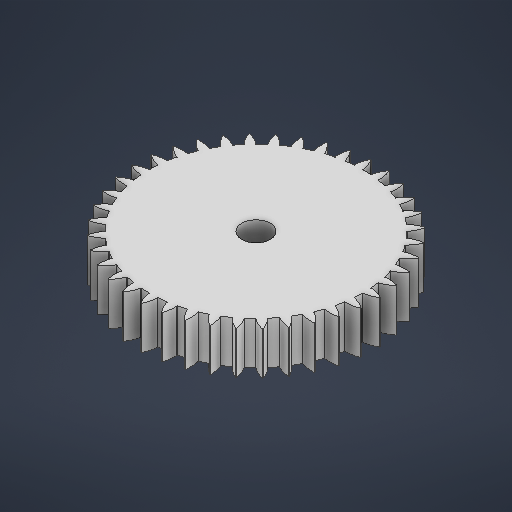
# Autodesk Inventor part: 80mm_40N_Gear
Saved by Autodesk Inventor 2026.2 (Build 302298000, 298)
## iProperties
Created: 2025-12-19
Part Number: 80mm_40N_Gear
Material: Generic
Document SubType Name: Modeling
Designer: Cobble
Density: 1 g/cm^3
Appearance: Default
Author: Cobble
Autodesk Inventor part; units mm, degrees
ref_plane "YZ Plane" through (0, 0, 0) normal (1, 0, 0) x (0, 1, 0)
ref_plane "XZ Plane" through (0, 0, 0) normal (0, 1, 0) x (-1, 0, 0)
ref_plane "XY Plane" through (0, 0, 0) normal (0, 0, 1) x (1, 0, 0)
sketch "Sketch1" plane through (0, 0, 0) normal (0, 0, 1) x (1, 0, 0)
  circle A0 centre (0, 0) radius 40
  circle A1 centre (0, 0) radius 42
  circle A2 centre (0, 0) radius 37.5
  circle A3 centre (0, 0) radius 37.5877 construction
  line L0 (0, 0) -> (0, 42) construction
  line L1 (0, 0) -> (-6.5702, 41.4829) construction
  line L2 (0, 0) -> (-12.9787, 39.9444) construction
  line L3 (0, 0) -> (-19.0676, 37.4223) construction
  line L4 (0, 0) -> (-24.687, 33.9787) construction
  line L5 (0, 0) -> (-29.6985, 29.6985) construction
  line L6 (0, 0) -> (-33.9787, 24.687) construction
  line L7 (0, 0) -> (-37.4223, 19.0676) construction
  line L8 (0, 0) -> (-39.9444, 12.9787) construction
  line L9 (0, 0) -> (-41.4829, 6.5702) construction
  line L10 (0, 0) -> (-42, 0) construction
  line L11 (0, 0) -> (-41.4829, -6.5702) construction
  line L12 (0, 0) -> (-39.9444, -12.9787) construction
  line L13 (0, 0) -> (-37.4223, -19.0676) construction
  line L14 (0, 0) -> (-33.9787, -24.687) construction
  line L15 (0, 0) -> (-29.6985, -29.6985) construction
  line L16 (0, 0) -> (-24.687, -33.9787) construction
  line L17 (0, 0) -> (-19.0676, -37.4223) construction
  line L18 (0, 0) -> (-12.9787, -39.9444) construction
  line L19 (0, 0) -> (-6.5702, -41.4829) construction
  line L20 (0, 0) -> (0, -42) construction
  line L21 (0, 0) -> (6.5702, -41.4829) construction
  line L22 (0, 0) -> (12.9787, -39.9444) construction
  line L23 (0, 0) -> (19.0676, -37.4223) construction
  line L24 (0, 0) -> (24.687, -33.9787) construction
  line L25 (0, 0) -> (29.6985, -29.6985) construction
  line L26 (0, 0) -> (33.9787, -24.687) construction
  line L27 (0, 0) -> (37.4223, -19.0676) construction
  line L28 (0, 0) -> (39.9444, -12.9787) construction
  line L29 (0, 0) -> (41.4829, -6.5702) construction
  line L30 (0, 0) -> (42, 0) construction
  line L31 (0, 0) -> (41.4829, 6.5702) construction
  line L32 (0, 0) -> (39.9444, 12.9787) construction
  line L33 (0, 0) -> (37.4223, 19.0676) construction
  line L34 (0, 0) -> (33.9787, 24.687) construction
  line L35 (0, 0) -> (29.6985, 29.6985) construction
  line L36 (0, 0) -> (24.687, 33.9787) construction
  line L37 (0, 0) -> (19.0676, 37.4223) construction
  line L38 (0, 0) -> (12.9787, 39.9444) construction
  line L39 (0, 0) -> (6.5702, 41.4829) construction
  line L40 (-5.88, 37.1249) -> (-0.0487, 38.0485) construction
  line L41 (-11.6152, 35.748) -> (-0.3852, 39.3969) construction
  line L42 (-17.0645, 33.4909) -> (-1.283, 41.532) construction
  line L43 (-22.0935, 30.4091) -> (-2.9878, 44.2902) construction
  line L44 (-26.5785, 26.5785) -> (-5.7047, 47.4523) construction
  line L45 (0, 0) -> (3.1384, 39.8767) construction
  line L46 (0, 0) -> (40, 0) construction
  line L47 (0, 0) -> (-3.1384, 39.8767) construction
  line L48 (0, 0) -> (-9.3378, 38.8948) construction
  line L49 (0, 0) -> (-15.3073, 36.9552) construction
  line L50 (0, 0) -> (-20.8999, 34.1056) construction
  line L51 (0, 0) -> (-25.9779, 30.4162) construction
  line L52 (0, 0) -> (-30.4162, 25.9779) construction
  line L53 (0, 0) -> (-34.1056, 20.8999) construction
  line L54 (0, 0) -> (-36.9552, 15.3073) construction
  line L55 (0, 0) -> (-38.8948, 9.3378) construction
  line L56 (0, 0) -> (-39.8767, 3.1384) construction
  line L57 (0, 0) -> (-39.8767, -3.1384) construction
  line L58 (0, 0) -> (-38.8948, -9.3378) construction
  line L59 (0, 0) -> (-36.9552, -15.3073) construction
  line L60 (0, 0) -> (-34.1056, -20.8999) construction
  line L61 (0, 0) -> (-30.4162, -25.9779) construction
  line L62 (0, 0) -> (-25.9779, -30.4162) construction
  line L63 (0, 0) -> (-20.8999, -34.1056) construction
  line L64 (0, 0) -> (-15.3073, -36.9552) construction
  line L65 (0, 0) -> (-9.3378, -38.8948) construction
  line L66 (0, 0) -> (-3.1384, -39.8767) construction
  line L67 (0, 0) -> (3.1384, -39.8767) construction
  line L68 (0, 0) -> (9.3378, -38.8948) construction
  line L69 (0, 0) -> (15.3073, -36.9552) construction
  line L70 (0, 0) -> (20.8999, -34.1056) construction
  line L71 (0, 0) -> (25.9779, -30.4162) construction
  line L72 (0, 0) -> (30.4162, -25.9779) construction
  line L73 (0, 0) -> (34.1056, -20.8999) construction
  line L74 (0, 0) -> (36.9552, -15.3073) construction
  line L75 (0, 0) -> (38.8948, -9.3378) construction
  line L76 (0, 0) -> (39.8767, -3.1384) construction
  line L77 (0, 0) -> (39.8767, 3.1384) construction
  line L78 (0, 0) -> (38.8948, 9.3378) construction
  line L79 (0, 0) -> (36.9552, 15.3073) construction
  line L80 (0, 0) -> (34.1056, 20.8999) construction
  line L81 (0, 0) -> (30.4162, 25.9779) construction
  line L82 (0, 0) -> (25.9779, 30.4162) construction
  line L83 (0, 0) -> (20.8999, 34.1056) construction
  line L84 (0, 0) -> (15.3073, 36.9552) construction
  line L85 (0, 0) -> (9.3378, 38.8948) construction
  line L86 (2.9491, 37.4718) -> (-2.9367, 37.9351) construction
  line L87 (8.7747, 36.5492) -> (-2.7071, 39.3057) construction
  line L88 (14.3842, 34.7265) -> (-1.9796, 41.5046) construction
  line L89 (19.6395, 32.0488) -> (-0.4964, 44.3881) construction
  line L90 (24.4113, 28.5819) -> (1.9641, 47.7536) construction
  spline S0 degree 4 poles (0, 37.5877) (0.0049, 37.8732) (-0.3682, 40.1269) (-1.7488, 42.8109) (-4.0108, 45.8093) (-5.7047, 47.4523) knots 0 0 0 0 0 0.384274 1 1 1 1 1
  spline S1 degree 4 poles (-2.9491, 37.4718) (-2.9764, 37.756) (-2.7812, 40.0321) (-1.6155, 42.8162) (0.4043, 45.9828) (1.9641, 47.7536) knots 0 0 0 0 0 0.384274 1 1 1 1 1
  line L91 (0, 37.5877) -> (0, 37.5)
  line L92 (-2.9491, 37.4718) -> (-2.9422, 37.3844)
  line L93 (-30.4091, 22.0935) -> (-13.0577, 45.9757) construction
  spline S2 degree 4 poles (-5.88, 37.1249) (-5.9198, 37.4076) (-6.6409, 39.5753) (-8.4244, 42.0103) (-11.1275, 44.6179) (-13.0577, 45.9757) knots 0 0 0 0 0 0.384274 1 1 1 1 1
  spline S3 degree 4 poles (-8.7747, 36.5492) (-8.8461, 36.8256) (-9.0094, 39.1042) (-8.2935, 42.0363) (-6.794, 45.4799) (-5.5304, 47.4729) knots 0 0 0 0 0 0.384274 1 1 1 1 1
  line L94 (-5.88, 37.1249) -> (-5.8663, 37.0383)
  line L95 (-8.7747, 36.5492) -> (-8.7542, 36.4639)
  line L96 (-33.4909, 17.0645) -> (-20.0891, 43.367) construction
  spline S4 degree 4 poles (-11.6152, 35.748) (-11.6988, 36.021) (-12.7501, 38.0492) (-14.8925, 40.1752) (-17.9703, 42.3278) (-20.0891, 43.367) knots 0 0 0 0 0 0.384274 1 1 1 1 1
  spline S5 degree 4 poles (-14.3842, 34.7265) (-14.4979, 34.9884) (-15.0157, 37.2134) (-14.7674, 40.2214) (-13.825, 43.8571) (-12.8887, 46.0233) knots 0 0 0 0 0 0.384274 1 1 1 1 1
  line L97 (-11.6152, 35.748) -> (-11.5881, 35.6646)
  line L98 (-14.3842, 34.7265) -> (-14.3506, 34.6455)
  line L99 (-35.748, 11.6152) -> (-26.6258, 39.6904) construction
  spline S6 degree 4 poles (-17.0645, 33.4909) (-17.1897, 33.7475) (-18.5453, 35.5862) (-20.9939, 37.3509) (-24.3706, 38.9955) (-26.6258, 39.6904) knots 0 0 0 0 0 0.384274 1 1 1 1 1
  spline S7 degree 4 poles (-19.6395, 32.0488) (-19.7928, 32.2896) (-20.6523, 34.4062) (-20.8776, 37.4161) (-20.5156, 41.1545) (-19.9297, 43.4405) knots 0 0 0 0 0 0.384274 1 1 1 1 1
  line L100 (-17.0645, 33.4909) -> (-17.0246, 33.4127)
  line L101 (-19.6395, 32.0488) -> (-19.5937, 31.974)
  line L102 (-37.1249, 5.88) -> (-32.507, 35.0366) construction
  spline S8 degree 4 poles (-22.0935, 30.4091) (-22.2573, 30.6429) (-23.8839, 32.2469) (-26.5784, 33.6069) (-30.1708, 34.703) (-32.507, 35.0366) knots 0 0 0 0 0 0.384274 1 1 1 1 1
  spline S9 degree 4 poles (-24.4113, 28.5819) (-24.6004, 28.7958) (-25.7803, 30.7519) (-26.4737, 33.6894) (-26.7009, 37.4385) (-26.4799, 39.7879) knots 0 0 0 0 0 0.384274 1 1 1 1 1
  line L103 (-22.0935, 30.4091) -> (-22.0419, 30.3381)
  line L104 (-24.4113, 28.5819) -> (-24.3543, 28.5152)
  line L105 (-37.5877, 0) -> (-37.5877, 29.52) construction
  spline S10 degree 4 poles (-26.5785, 26.5785) (-26.7769, 26.7838) (-28.6344, 28.1136) (-31.5085, 29.0353) (-35.2281, 29.556) (-37.5877, 29.52) knots 0 0 0 0 0 0.384274 1 1 1 1 1
  spline S11 degree 4 poles (-28.5819, 24.4113) (-28.8022, 24.5929) (-30.2736, 26.3404) (-31.4179, 29.1333) (-32.2289, 32.8006) (-32.3781, 35.1557) knots 0 0 0 0 0 0.384274 1 1 1 1 1
  line L106 (-26.5785, 26.5785) -> (-26.5165, 26.5165)
  line L107 (-28.5819, 24.4113) -> (-28.5152, 24.3543)
  line L108 (-37.1249, -5.88) -> (-41.7429, 23.2765) construction
  spline S12 degree 4 poles (-30.4091, 22.0935) (-30.6372, 22.2652) (-32.6798, 23.2881) (-35.6627, 23.7488) (-39.418, 23.6813) (-41.7429, 23.2765) knots 0 0 0 0 0 0.384274 1 1 1 1 1
  spline S13 degree 4 poles (-32.0488, 19.6395) (-32.2947, 19.7845) (-34.0214, 21.2802) (-35.5886, 23.8597) (-36.9632, 27.355) (-37.479, 29.6578) knots 0 0 0 0 0 0.384274 1 1 1 1 1
  line L109 (-30.4091, 22.0935) -> (-30.3381, 22.0419)
  line L110 (-32.0488, 19.6395) -> (-31.974, 19.5937)
  line L111 (-35.748, -11.6152) -> (-44.8702, 16.4599) construction
  spline S14 degree 4 poles (-33.4909, 17.0645) (-33.743, 17.1984) (-35.9205, 17.8891) (-38.9388, 17.8776) (-42.6372, 17.2234) (-44.8702, 16.4599) knots 0 0 0 0 0 0.384274 1 1 1 1 1
  spline S15 degree 4 poles (-34.7265, 14.3842) (-34.9921, 14.4889) (-36.9315, 15.6961) (-38.8829, 17.9987) (-40.7874, 21.2359) (-41.6571, 23.4297) knots 0 0 0 0 0 0.384274 1 1 1 1 1
  line L112 (-33.4909, 17.0645) -> (-33.4127, 17.0246)
  line L113 (-34.7265, 14.3842) -> (-34.6455, 14.3506)
  line L114 (-33.4909, -17.0645) -> (-46.8927, 9.2381) construction
  spline S16 degree 4 poles (-35.748, 11.6152) (-36.018, 11.7081) (-38.2768, 12.0497) (-41.256, 11.5661) (-44.8066, 10.3414) (-46.8927, 9.2381) knots 0 0 0 0 0 0.384274 1 1 1 1 1
  spline S17 degree 4 poles (-36.5492, 8.7747) (-36.8279, 8.8366) (-38.9322, 9.7255) (-41.2198, 11.6945) (-43.6073, 14.5939) (-44.8095, 16.6246) knots 0 0 0 0 0 0.384274 1 1 1 1 1
  line L115 (-35.748, 11.6152) -> (-35.6646, 11.5881)
  line L116 (-36.5492, 8.7747) -> (-36.4639, 8.7542)
  line L117 (-30.4091, -22.0935) -> (-47.7605, 1.7887) construction
  spline S18 degree 4 poles (-37.1249, 5.88) (-37.4061, 5.9295) (-39.6905, 5.9135) (-42.5574, 4.9699) (-45.8727, 3.2048) (-47.7605, 1.7887) knots 0 0 0 0 0 0.384274 1 1 1 1 1
  spline S19 degree 4 poles (-37.4718, 2.9491) (-37.7568, 2.9666) (-39.9743, 3.5154) (-42.5418, 5.1023) (-45.3534, 7.5926) (-46.8584, 9.4102) knots 0 0 0 0 0 0.384274 1 1 1 1 1
  line L118 (-37.1249, 5.88) -> (-37.0383, 5.8663)
  line L119 (-37.4718, 2.9491) -> (-37.3844, 2.9422)
  line L120 (-26.5785, -26.5785) -> (-47.4523, -5.7047) construction
  spline S20 degree 4 poles (-37.5877, 0) (-37.8732, 0.0049) (-40.1269, -0.3682) (-42.8109, -1.7488) (-45.8093, -4.0108) (-47.4523, -5.7047) knots 0 0 0 0 0 0.384274 1 1 1 1 1
  spline S21 degree 4 poles (-37.4718, -2.9491) (-37.756, -2.9764) (-40.0321, -2.7812) (-42.8162, -1.6155) (-45.9828, 0.4043) (-47.7536, 1.9641) knots 0 0 0 0 0 0.384274 1 1 1 1 1
  line L121 (-37.5877, 0) -> (-37.5, 0)
  line L122 (-37.4718, -2.9491) -> (-37.3844, -2.9422)
  line L123 (-22.0935, -30.4091) -> (-45.9757, -13.0577) construction
  spline S22 degree 4 poles (-37.1249, -5.88) (-37.4076, -5.9198) (-39.5753, -6.6409) (-42.0103, -8.4244) (-44.6179, -11.1275) (-45.9757, -13.0577) knots 0 0 0 0 0 0.384274 1 1 1 1 1
  spline S23 degree 4 poles (-36.5492, -8.7747) (-36.8256, -8.8461) (-39.1042, -9.0094) (-42.0363, -8.2935) (-45.4799, -6.794) (-47.4729, -5.5304) knots 0 0 0 0 0 0.384274 1 1 1 1 1
  line L124 (-37.1249, -5.88) -> (-37.0383, -5.8663)
  line L125 (-36.5492, -8.7747) -> (-36.4639, -8.7542)
  line L126 (-17.0645, -33.4909) -> (-43.367, -20.0891) construction
  spline S24 degree 4 poles (-35.748, -11.6152) (-36.021, -11.6988) (-38.0492, -12.7501) (-40.1752, -14.8925) (-42.3278, -17.9703) (-43.367, -20.0891) knots 0 0 0 0 0 0.384274 1 1 1 1 1
  spline S25 degree 4 poles (-34.7265, -14.3842) (-34.9884, -14.4979) (-37.2134, -15.0157) (-40.2214, -14.7674) (-43.8571, -13.825) (-46.0233, -12.8887) knots 0 0 0 0 0 0.384274 1 1 1 1 1
  line L127 (-35.748, -11.6152) -> (-35.6646, -11.5881)
  line L128 (-34.7265, -14.3842) -> (-34.6455, -14.3506)
  line L129 (-11.6152, -35.748) -> (-39.6904, -26.6258) construction
  spline S26 degree 4 poles (-33.4909, -17.0645) (-33.7475, -17.1897) (-35.5862, -18.5453) (-37.3509, -20.9939) (-38.9955, -24.3706) (-39.6904, -26.6258) knots 0 0 0 0 0 0.384274 1 1 1 1 1
  spline S27 degree 4 poles (-32.0488, -19.6395) (-32.2896, -19.7928) (-34.4062, -20.6523) (-37.4161, -20.8776) (-41.1545, -20.5156) (-43.4405, -19.9297) knots 0 0 0 0 0 0.384274 1 1 1 1 1
  line L130 (-33.4909, -17.0645) -> (-33.4127, -17.0246)
  line L131 (-32.0488, -19.6395) -> (-31.974, -19.5937)
  line L132 (-5.88, -37.1249) -> (-35.0366, -32.507) construction
  spline S28 degree 4 poles (-30.4091, -22.0935) (-30.6429, -22.2573) (-32.2469, -23.8839) (-33.6069, -26.5784) (-34.703, -30.1708) (-35.0366, -32.507) knots 0 0 0 0 0 0.384274 1 1 1 1 1
  spline S29 degree 4 poles (-28.5819, -24.4113) (-28.7958, -24.6004) (-30.7519, -25.7803) (-33.6894, -26.4737) (-37.4385, -26.7009) (-39.7879, -26.4799) knots 0 0 0 0 0 0.384274 1 1 1 1 1
  line L133 (-30.4091, -22.0935) -> (-30.3381, -22.0419)
  line L134 (-28.5819, -24.4113) -> (-28.5152, -24.3543)
  line L135 (0, -37.5877) -> (-29.52, -37.5877) construction
  spline S30 degree 4 poles (-26.5785, -26.5785) (-26.7838, -26.7769) (-28.1136, -28.6344) (-29.0353, -31.5085) (-29.556, -35.2281) (-29.52, -37.5877) knots 0 0 0 0 0 0.384274 1 1 1 1 1
  spline S31 degree 4 poles (-24.4113, -28.5819) (-24.5929, -28.8022) (-26.3404, -30.2736) (-29.1333, -31.4179) (-32.8006, -32.2289) (-35.1557, -32.3781) knots 0 0 0 0 0 0.384274 1 1 1 1 1
  line L136 (-26.5785, -26.5785) -> (-26.5165, -26.5165)
  line L137 (-24.4113, -28.5819) -> (-24.3543, -28.5152)
  line L138 (5.88, -37.1249) -> (-23.2765, -41.7429) construction
  spline S32 degree 4 poles (-22.0935, -30.4091) (-22.2652, -30.6372) (-23.2881, -32.6798) (-23.7488, -35.6627) (-23.6813, -39.418) (-23.2765, -41.7429) knots 0 0 0 0 0 0.384274 1 1 1 1 1
  spline S33 degree 4 poles (-19.6395, -32.0488) (-19.7845, -32.2947) (-21.2802, -34.0214) (-23.8597, -35.5886) (-27.355, -36.9632) (-29.6578, -37.479) knots 0 0 0 0 0 0.384274 1 1 1 1 1
  line L139 (-22.0935, -30.4091) -> (-22.0419, -30.3381)
  line L140 (-19.6395, -32.0488) -> (-19.5937, -31.974)
  line L141 (11.6152, -35.748) -> (-16.4599, -44.8702) construction
  spline S34 degree 4 poles (-17.0645, -33.4909) (-17.1984, -33.743) (-17.8891, -35.9205) (-17.8776, -38.9388) (-17.2234, -42.6372) (-16.4599, -44.8702) knots 0 0 0 0 0 0.384274 1 1 1 1 1
  spline S35 degree 4 poles (-14.3842, -34.7265) (-14.4889, -34.9921) (-15.6961, -36.9315) (-17.9987, -38.8829) (-21.2359, -40.7874) (-23.4297, -41.6571) knots 0 0 0 0 0 0.384274 1 1 1 1 1
  line L142 (-17.0645, -33.4909) -> (-17.0246, -33.4127)
  line L143 (-14.3842, -34.7265) -> (-14.3506, -34.6455)
  line L144 (17.0645, -33.4909) -> (-9.2381, -46.8927) construction
  spline S36 degree 4 poles (-11.6152, -35.748) (-11.7081, -36.018) (-12.0497, -38.2768) (-11.5661, -41.256) (-10.3414, -44.8066) (-9.2381, -46.8927) knots 0 0 0 0 0 0.384274 1 1 1 1 1
  spline S37 degree 4 poles (-8.7747, -36.5492) (-8.8366, -36.8279) (-9.7255, -38.9322) (-11.6945, -41.2198) (-14.5939, -43.6073) (-16.6246, -44.8095) knots 0 0 0 0 0 0.384274 1 1 1 1 1
  line L145 (-11.6152, -35.748) -> (-11.5881, -35.6646)
  line L146 (-8.7747, -36.5492) -> (-8.7542, -36.4639)
  line L147 (22.0935, -30.4091) -> (-1.7887, -47.7605) construction
  spline S38 degree 4 poles (-5.88, -37.1249) (-5.9295, -37.4061) (-5.9135, -39.6905) (-4.9699, -42.5574) (-3.2048, -45.8727) (-1.7887, -47.7605) knots 0 0 0 0 0 0.384274 1 1 1 1 1
  spline S39 degree 4 poles (-2.9491, -37.4718) (-2.9666, -37.7568) (-3.5154, -39.9743) (-5.1023, -42.5418) (-7.5926, -45.3534) (-9.4102, -46.8584) knots 0 0 0 0 0 0.384274 1 1 1 1 1
  line L148 (-5.88, -37.1249) -> (-5.8663, -37.0383)
  line L149 (-2.9491, -37.4718) -> (-2.9422, -37.3844)
  line L150 (26.5785, -26.5785) -> (5.7047, -47.4523) construction
  spline S40 degree 4 poles (0, -37.5877) (-0.0049, -37.8732) (0.3682, -40.1269) (1.7488, -42.8109) (4.0108, -45.8093) (5.7047, -47.4523) knots 0 0 0 0 0 0.384274 1 1 1 1 1
  spline S41 degree 4 poles (2.9491, -37.4718) (2.9764, -37.756) (2.7812, -40.0321) (1.6155, -42.8162) (-0.4043, -45.9828) (-1.9641, -47.7536) knots 0 0 0 0 0 0.384274 1 1 1 1 1
  line L151 (0, -37.5877) -> (0, -37.5)
  line L152 (2.9491, -37.4718) -> (2.9422, -37.3844)
  line L153 (30.4091, -22.0935) -> (13.0577, -45.9757) construction
  spline S42 degree 4 poles (5.88, -37.1249) (5.9198, -37.4076) (6.6409, -39.5753) (8.4244, -42.0103) (11.1275, -44.6179) (13.0577, -45.9757) knots 0 0 0 0 0 0.384274 1 1 1 1 1
  spline S43 degree 4 poles (8.7747, -36.5492) (8.8461, -36.8256) (9.0094, -39.1042) (8.2935, -42.0363) (6.794, -45.4799) (5.5304, -47.4729) knots 0 0 0 0 0 0.384274 1 1 1 1 1
  line L154 (5.88, -37.1249) -> (5.8663, -37.0383)
  line L155 (8.7747, -36.5492) -> (8.7542, -36.4639)
  line L156 (33.4909, -17.0645) -> (20.0891, -43.367) construction
  spline S44 degree 4 poles (11.6152, -35.748) (11.6988, -36.021) (12.7501, -38.0492) (14.8925, -40.1752) (17.9703, -42.3278) (20.0891, -43.367) knots 0 0 0 0 0 0.384274 1 1 1 1 1
  spline S45 degree 4 poles (14.3842, -34.7265) (14.4979, -34.9884) (15.0157, -37.2134) (14.7674, -40.2214) (13.825, -43.8571) (12.8887, -46.0233) knots 0 0 0 0 0 0.384274 1 1 1 1 1
  line L157 (11.6152, -35.748) -> (11.5881, -35.6646)
  line L158 (14.3842, -34.7265) -> (14.3506, -34.6455)
  line L159 (35.748, -11.6152) -> (26.6258, -39.6904) construction
  spline S46 degree 4 poles (17.0645, -33.4909) (17.1897, -33.7475) (18.5453, -35.5862) (20.9939, -37.3509) (24.3706, -38.9955) (26.6258, -39.6904) knots 0 0 0 0 0 0.384274 1 1 1 1 1
  spline S47 degree 4 poles (19.6395, -32.0488) (19.7928, -32.2896) (20.6523, -34.4062) (20.8776, -37.4161) (20.5156, -41.1545) (19.9297, -43.4405) knots 0 0 0 0 0 0.384274 1 1 1 1 1
  line L160 (17.0645, -33.4909) -> (17.0246, -33.4127)
  line L161 (19.6395, -32.0488) -> (19.5937, -31.974)
  line L162 (37.1249, -5.88) -> (32.507, -35.0366) construction
  spline S48 degree 4 poles (22.0935, -30.4091) (22.2573, -30.6429) (23.8839, -32.2469) (26.5784, -33.6069) (30.1708, -34.703) (32.507, -35.0366) knots 0 0 0 0 0 0.384274 1 1 1 1 1
  spline S49 degree 4 poles (24.4113, -28.5819) (24.6004, -28.7958) (25.7803, -30.7519) (26.4737, -33.6894) (26.7009, -37.4385) (26.4799, -39.7879) knots 0 0 0 0 0 0.384274 1 1 1 1 1
  line L163 (22.0935, -30.4091) -> (22.0419, -30.3381)
  line L164 (24.4113, -28.5819) -> (24.3543, -28.5152)
  line L165 (37.5877, 0) -> (37.5877, -29.52) construction
  spline S50 degree 4 poles (26.5785, -26.5785) (26.7769, -26.7838) (28.6344, -28.1136) (31.5085, -29.0353) (35.2281, -29.556) (37.5877, -29.52) knots 0 0 0 0 0 0.384274 1 1 1 1 1
  spline S51 degree 4 poles (28.5819, -24.4113) (28.8022, -24.5929) (30.2736, -26.3404) (31.4179, -29.1333) (32.2289, -32.8006) (32.3781, -35.1557) knots 0 0 0 0 0 0.384274 1 1 1 1 1
  line L166 (26.5785, -26.5785) -> (26.5165, -26.5165)
  line L167 (28.5819, -24.4113) -> (28.5152, -24.3543)
  line L168 (37.1249, 5.88) -> (41.7429, -23.2765) construction
  spline S52 degree 4 poles (30.4091, -22.0935) (30.6372, -22.2652) (32.6798, -23.2881) (35.6627, -23.7488) (39.418, -23.6813) (41.7429, -23.2765) knots 0 0 0 0 0 0.384274 1 1 1 1 1
  spline S53 degree 4 poles (32.0488, -19.6395) (32.2947, -19.7845) (34.0214, -21.2802) (35.5886, -23.8597) (36.9632, -27.355) (37.479, -29.6578) knots 0 0 0 0 0 0.384274 1 1 1 1 1
  line L169 (30.4091, -22.0935) -> (30.3381, -22.0419)
  line L170 (32.0488, -19.6395) -> (31.974, -19.5937)
  line L171 (35.748, 11.6152) -> (44.8702, -16.4599) construction
  spline S54 degree 4 poles (33.4909, -17.0645) (33.743, -17.1984) (35.9205, -17.8891) (38.9388, -17.8776) (42.6372, -17.2234) (44.8702, -16.4599) knots 0 0 0 0 0 0.384274 1 1 1 1 1
  spline S55 degree 4 poles (34.7265, -14.3842) (34.9921, -14.4889) (36.9315, -15.6961) (38.8829, -17.9987) (40.7874, -21.2359) (41.6571, -23.4297) knots 0 0 0 0 0 0.384274 1 1 1 1 1
  line L172 (33.4909, -17.0645) -> (33.4127, -17.0246)
  line L173 (34.7265, -14.3842) -> (34.6455, -14.3506)
  line L174 (33.4909, 17.0645) -> (46.8927, -9.2381) construction
  spline S56 degree 4 poles (35.748, -11.6152) (36.018, -11.7081) (38.2768, -12.0497) (41.256, -11.5661) (44.8066, -10.3414) (46.8927, -9.2381) knots 0 0 0 0 0 0.384274 1 1 1 1 1
  spline S57 degree 4 poles (36.5492, -8.7747) (36.8279, -8.8366) (38.9322, -9.7255) (41.2198, -11.6945) (43.6073, -14.5939) (44.8095, -16.6246) knots 0 0 0 0 0 0.384274 1 1 1 1 1
  line L175 (35.748, -11.6152) -> (35.6646, -11.5881)
  line L176 (36.5492, -8.7747) -> (36.4639, -8.7542)
  line L177 (30.4091, 22.0935) -> (47.7605, -1.7887) construction
  spline S58 degree 4 poles (37.1249, -5.88) (37.4061, -5.9295) (39.6905, -5.9135) (42.5574, -4.9699) (45.8727, -3.2048) (47.7605, -1.7887) knots 0 0 0 0 0 0.384274 1 1 1 1 1
  spline S59 degree 4 poles (37.4718, -2.9491) (37.7568, -2.9666) (39.9743, -3.5154) (42.5418, -5.1023) (45.3534, -7.5926) (46.8584, -9.4102) knots 0 0 0 0 0 0.384274 1 1 1 1 1
  line L178 (37.1249, -5.88) -> (37.0383, -5.8663)
  line L179 (37.4718, -2.9491) -> (37.3844, -2.9422)
  line L180 (26.5785, 26.5785) -> (47.4523, 5.7047) construction
  spline S60 degree 4 poles (37.5877, 0) (37.8732, -0.0049) (40.1269, 0.3682) (42.8109, 1.7488) (45.8093, 4.0108) (47.4523, 5.7047) knots 0 0 0 0 0 0.384274 1 1 1 1 1
  spline S61 degree 4 poles (37.4718, 2.9491) (37.756, 2.9764) (40.0321, 2.7812) (42.8162, 1.6155) (45.9828, -0.4043) (47.7536, -1.9641) knots 0 0 0 0 0 0.384274 1 1 1 1 1
  line L181 (37.5877, 0) -> (37.5, 0)
  line L182 (37.4718, 2.9491) -> (37.3844, 2.9422)
  line L183 (22.0935, 30.4091) -> (45.9757, 13.0577) construction
  spline S62 degree 4 poles (37.1249, 5.88) (37.4076, 5.9198) (39.5753, 6.6409) (42.0103, 8.4244) (44.6179, 11.1275) (45.9757, 13.0577) knots 0 0 0 0 0 0.384274 1 1 1 1 1
  spline S63 degree 4 poles (36.5492, 8.7747) (36.8256, 8.8461) (39.1042, 9.0094) (42.0363, 8.2935) (45.4799, 6.794) (47.4729, 5.5304) knots 0 0 0 0 0 0.384274 1 1 1 1 1
  line L184 (37.1249, 5.88) -> (37.0383, 5.8663)
  line L185 (36.5492, 8.7747) -> (36.4639, 8.7542)
  line L186 (17.0645, 33.4909) -> (43.367, 20.0891) construction
  spline S64 degree 4 poles (35.748, 11.6152) (36.021, 11.6988) (38.0492, 12.7501) (40.1752, 14.8925) (42.3278, 17.9703) (43.367, 20.0891) knots 0 0 0 0 0 0.384274 1 1 1 1 1
  spline S65 degree 4 poles (34.7265, 14.3842) (34.9884, 14.4979) (37.2134, 15.0157) (40.2214, 14.7674) (43.8571, 13.825) (46.0233, 12.8887) knots 0 0 0 0 0 0.384274 1 1 1 1 1
  line L187 (35.748, 11.6152) -> (35.6646, 11.5881)
  line L188 (34.7265, 14.3842) -> (34.6455, 14.3506)
  line L189 (11.6152, 35.748) -> (39.6904, 26.6258) construction
  spline S66 degree 4 poles (33.4909, 17.0645) (33.7475, 17.1897) (35.5862, 18.5453) (37.3509, 20.9939) (38.9955, 24.3706) (39.6904, 26.6258) knots 0 0 0 0 0 0.384274 1 1 1 1 1
  spline S67 degree 4 poles (32.0488, 19.6395) (32.2896, 19.7928) (34.4062, 20.6523) (37.4161, 20.8776) (41.1545, 20.5156) (43.4405, 19.9297) knots 0 0 0 0 0 0.384274 1 1 1 1 1
  line L190 (33.4909, 17.0645) -> (33.4127, 17.0246)
  line L191 (32.0488, 19.6395) -> (31.974, 19.5937)
  line L192 (5.88, 37.1249) -> (35.0366, 32.507) construction
  spline S68 degree 4 poles (30.4091, 22.0935) (30.6429, 22.2573) (32.2469, 23.8839) (33.6069, 26.5784) (34.703, 30.1708) (35.0366, 32.507) knots 0 0 0 0 0 0.384274 1 1 1 1 1
  spline S69 degree 4 poles (28.5819, 24.4113) (28.7958, 24.6004) (30.7519, 25.7803) (33.6894, 26.4737) (37.4385, 26.7009) (39.7879, 26.4799) knots 0 0 0 0 0 0.384274 1 1 1 1 1
  line L193 (30.4091, 22.0935) -> (30.3381, 22.0419)
  line L194 (28.5819, 24.4113) -> (28.5152, 24.3543)
  line L195 (0, 37.5877) -> (29.52, 37.5877) construction
  spline S70 degree 4 poles (26.5785, 26.5785) (26.7838, 26.7769) (28.1136, 28.6344) (29.0353, 31.5085) (29.556, 35.2281) (29.52, 37.5877) knots 0 0 0 0 0 0.384274 1 1 1 1 1
  spline S71 degree 4 poles (24.4113, 28.5819) (24.5929, 28.8022) (26.3404, 30.2736) (29.1333, 31.4179) (32.8006, 32.2289) (35.1557, 32.3781) knots 0 0 0 0 0 0.384274 1 1 1 1 1
  line L196 (26.5785, 26.5785) -> (26.5165, 26.5165)
  line L197 (24.4113, 28.5819) -> (24.3543, 28.5152)
  line L198 (-5.88, 37.1249) -> (23.2765, 41.7429) construction
  spline S72 degree 4 poles (22.0935, 30.4091) (22.2652, 30.6372) (23.2881, 32.6798) (23.7488, 35.6627) (23.6813, 39.418) (23.2765, 41.7429) knots 0 0 0 0 0 0.384274 1 1 1 1 1
  spline S73 degree 4 poles (19.6395, 32.0488) (19.7845, 32.2947) (21.2802, 34.0214) (23.8597, 35.5886) (27.355, 36.9632) (29.6578, 37.479) knots 0 0 0 0 0 0.384274 1 1 1 1 1
  line L199 (22.0935, 30.4091) -> (22.0419, 30.3381)
  line L200 (19.6395, 32.0488) -> (19.5937, 31.974)
  line L201 (-11.6152, 35.748) -> (16.4599, 44.8702) construction
  spline S74 degree 4 poles (17.0645, 33.4909) (17.1984, 33.743) (17.8891, 35.9205) (17.8776, 38.9388) (17.2234, 42.6372) (16.4599, 44.8702) knots 0 0 0 0 0 0.384274 1 1 1 1 1
  spline S75 degree 4 poles (14.3842, 34.7265) (14.4889, 34.9921) (15.6961, 36.9315) (17.9987, 38.8829) (21.2359, 40.7874) (23.4297, 41.6571) knots 0 0 0 0 0 0.384274 1 1 1 1 1
  line L202 (17.0645, 33.4909) -> (17.0246, 33.4127)
  line L203 (14.3842, 34.7265) -> (14.3506, 34.6455)
  line L204 (-17.0645, 33.4909) -> (9.2381, 46.8927) construction
  spline S76 degree 4 poles (11.6152, 35.748) (11.7081, 36.018) (12.0497, 38.2768) (11.5661, 41.256) (10.3414, 44.8066) (9.2381, 46.8927) knots 0 0 0 0 0 0.384274 1 1 1 1 1
  spline S77 degree 4 poles (8.7747, 36.5492) (8.8366, 36.8279) (9.7255, 38.9322) (11.6945, 41.2198) (14.5939, 43.6073) (16.6246, 44.8095) knots 0 0 0 0 0 0.384274 1 1 1 1 1
  line L205 (11.6152, 35.748) -> (11.5881, 35.6646)
  line L206 (8.7747, 36.5492) -> (8.7542, 36.4639)
  line L207 (-22.0935, 30.4091) -> (1.7887, 47.7605) construction
  spline S78 degree 4 poles (5.88, 37.1249) (5.9295, 37.4061) (5.9135, 39.6905) (4.9699, 42.5574) (3.2048, 45.8727) (1.7887, 47.7605) knots 0 0 0 0 0 0.384274 1 1 1 1 1
  spline S79 degree 4 poles (2.9491, 37.4718) (2.9666, 37.7568) (3.5154, 39.9743) (5.1023, 42.5418) (7.5926, 45.3534) (9.4102, 46.8584) knots 0 0 0 0 0 0.384274 1 1 1 1 1
  line L208 (5.88, 37.1249) -> (5.8663, 37.0383)
  line L209 (2.9491, 37.4718) -> (2.9422, 37.3844)
  point P0 (-6.0002, 37.5725)
  point P1 (-6.5435, 38.8516)
  point P2 (-7.7642, 40.8199)
  point P3 (-9.8795, 43.2776)
  point P4 (-8.8349, 37.0086)
  point P5 (-8.8225, 38.3983)
  point P6 (-8.4479, 40.6839)
  point P7 (-7.4341, 43.764)
  point P8 (-11.804, 36.1713)
  point P9 (-12.5406, 37.3497)
  point P10 (-14.0542, 39.1028)
  point P11 (-16.528, 41.1992)
  point P12 (-14.5155, 35.1709)
  point P13 (-14.7207, 36.5454)
  point P14 (-14.7083, 38.8615)
  point P15 (-14.1888, 42.0622)
  point P16 (-17.3171, 33.8794)
  point P17 (-18.229, 34.928)
  point P18 (-19.9982, 36.4228)
  point P19 (-22.7695, 38.1065)
  point P20 (-19.8388, 32.4671)
  point P21 (-20.2564, 33.7926)
  point P22 (-20.6065, 36.0822)
  point P23 (-20.5941, 39.3247)
  point P24 (-22.4038, 30.7533)
  point P25 (-23.4685, 31.6464)
  point P26 (-25.4498, 32.846)
  point P27 (-28.4503, 34.0754)
  point P28 (-24.6735, 28.964)
  point P29 (-25.2934, 30.2078)
  point P30 (-25.9973, 32.4144)
  point P31 (-26.4923, 35.6189)
  point P32 (-26.9388, 26.8699)
  point P33 (-28.1302, 27.5855)
  point P34 (-30.2747, 28.4604)
  point P35 (-33.4306, 29.2053)
  point P36 (-28.9007, 24.7476)
  point P37 (-29.7075, 25.8791)
  point P38 (-30.7479, 27.9484)
  point P39 (-31.7382, 31.0361)
  point P40 (-30.8105, 22.325)
  point P41 (-32.0992, 22.8453)
  point P42 (-34.3542, 23.3739)
  point P43 (-37.5877, 23.616)
  point P44 (-32.4163, 19.9218)
  point P45 (-33.3901, 20.9132)
  point P46 (-34.7415, 22.7943)
  point P47 (-36.2025, 25.6891)
  point P48 (-33.9236, 17.2303)
  point P49 (-35.2778, 17.5426)
  point P50 (-37.5877, 17.712)
  point P51 (-40.8193, 17.4452)
  point P52 (-35.1336, 14.6055)
  point P53 (-36.2506, 15.4324)
  point P54 (-37.8796, 17.0789)
  point P55 (-39.7755, 19.7095)
  point P56 (-36.2013, 11.7113)
  point P57 (-37.5877, 11.808)
  point P58 (-39.8957, 11.6139)
  point P59 (-43.0458, 10.8449)
  point P60 (-36.9859, 8.9296)
  point P61 (-38.2184, 9.5715)
  point P62 (-40.0849, 10.943)
  point P63 (-42.369, 13.2445)
  point P64 (-37.5877, 5.904)
  point P65 (-38.9721, 5.7826)
  point P66 (-41.2213, 5.2299)
  point P67 (-44.2123, 3.9775)
  point P68 (-37.9274, 3.0338)
  point P69 (-39.2452, 3.475)
  point P70 (-41.3033, 4.5376)
  point P71 (-43.9193, 6.4535)
  point P72 (-38.0485, -0.0487)
  point P73 (-39.3969, -0.3852)
  point P74 (-41.532, -1.283)
  point P75 (-44.2902, -2.9878)
  point P76 (-37.9351, -2.9367)
  point P77 (-39.3057, -2.7071)
  point P78 (-41.5046, -1.9796)
  point P79 (-44.3881, -0.4964)
  point P80 (-37.5725, -6.0002)
  point P81 (-38.8516, -6.5435)
  point P82 (-40.8199, -7.7642)
  point P83 (-43.2776, -9.8795)
  point P84 (-37.0086, -8.8349)
  point P85 (-38.3983, -8.8225)
  point P86 (-40.6839, -8.4479)
  point P87 (-43.764, -7.4341)
  point P88 (-36.1713, -11.804)
  point P89 (-37.3497, -12.5406)
  point P90 (-39.1028, -14.0542)
  point P91 (-41.1992, -16.528)
  point P92 (-35.1709, -14.5155)
  point P93 (-36.5454, -14.7207)
  point P94 (-38.8615, -14.7083)
  point P95 (-42.0622, -14.1888)
  point P96 (-33.8794, -17.3171)
  point P97 (-34.928, -18.229)
  point P98 (-36.4228, -19.9982)
  point P99 (-38.1065, -22.7695)
  point P100 (-32.4671, -19.8388)
  point P101 (-33.7926, -20.2564)
  point P102 (-36.0822, -20.6065)
  point P103 (-39.3247, -20.5941)
  point P104 (-30.7533, -22.4038)
  point P105 (-31.6464, -23.4685)
  point P106 (-32.846, -25.4498)
  point P107 (-34.0754, -28.4503)
  point P108 (-28.964, -24.6735)
  point P109 (-30.2078, -25.2934)
  point P110 (-32.4144, -25.9973)
  point P111 (-35.6189, -26.4923)
  point P112 (-26.8699, -26.9388)
  point P113 (-27.5855, -28.1302)
  point P114 (-28.4604, -30.2747)
  point P115 (-29.2053, -33.4306)
  point P116 (-24.7476, -28.9007)
  point P117 (-25.8791, -29.7075)
  point P118 (-27.9484, -30.7479)
  point P119 (-31.0361, -31.7382)
  point P120 (-22.325, -30.8105)
  point P121 (-22.8453, -32.0992)
  point P122 (-23.3739, -34.3542)
  point P123 (-23.616, -37.5877)
  point P124 (-19.9218, -32.4163)
  point P125 (-20.9132, -33.3901)
  point P126 (-22.7943, -34.7415)
  point P127 (-25.6891, -36.2025)
  point P128 (-17.2303, -33.9236)
  point P129 (-17.5426, -35.2778)
  point P130 (-17.712, -37.5877)
  point P131 (-17.4452, -40.8193)
  point P132 (-14.6055, -35.1336)
  point P133 (-15.4324, -36.2506)
  point P134 (-17.0789, -37.8796)
  point P135 (-19.7095, -39.7755)
  point P136 (-11.7113, -36.2013)
  point P137 (-11.808, -37.5877)
  point P138 (-11.6139, -39.8957)
  point P139 (-10.8449, -43.0458)
  point P140 (-8.9296, -36.9859)
  point P141 (-9.5715, -38.2184)
  point P142 (-10.943, -40.0849)
  point P143 (-13.2445, -42.369)
  point P144 (-5.904, -37.5877)
  point P145 (-5.7826, -38.9721)
  point P146 (-5.2299, -41.2213)
  point P147 (-3.9775, -44.2123)
  point P148 (-3.0338, -37.9274)
  point P149 (-3.475, -39.2452)
  point P150 (-4.5376, -41.3033)
  point P151 (-6.4535, -43.9193)
  point P152 (0.0487, -38.0485)
  point P153 (0.3852, -39.3969)
  point P154 (1.283, -41.532)
  point P155 (2.9878, -44.2902)
  point P156 (2.9367, -37.9351)
  point P157 (2.7071, -39.3057)
  point P158 (1.9796, -41.5046)
  point P159 (0.4964, -44.3881)
  point P160 (6.0002, -37.5725)
  point P161 (6.5435, -38.8516)
  point P162 (7.7642, -40.8199)
  point P163 (9.8795, -43.2776)
  point P164 (8.8349, -37.0086)
  point P165 (8.8225, -38.3983)
  point P166 (8.4479, -40.6839)
  point P167 (7.4341, -43.764)
  point P168 (11.804, -36.1713)
  point P169 (12.5406, -37.3497)
  point P170 (14.0542, -39.1028)
  point P171 (16.528, -41.1992)
  point P172 (14.5155, -35.1709)
  point P173 (14.7207, -36.5454)
  point P174 (14.7083, -38.8615)
  point P175 (14.1888, -42.0622)
  point P176 (17.3171, -33.8794)
  point P177 (18.229, -34.928)
  point P178 (19.9982, -36.4228)
  point P179 (22.7695, -38.1065)
  point P180 (19.8388, -32.4671)
  point P181 (20.2564, -33.7926)
  point P182 (20.6065, -36.0822)
  point P183 (20.5941, -39.3247)
  point P184 (22.4038, -30.7533)
  point P185 (23.4685, -31.6464)
  point P186 (25.4498, -32.846)
  point P187 (28.4503, -34.0754)
  point P188 (24.6735, -28.964)
  point P189 (25.2934, -30.2078)
  point P190 (25.9973, -32.4144)
  point P191 (26.4923, -35.6189)
  point P192 (26.9388, -26.8699)
  point P193 (28.1302, -27.5855)
  point P194 (30.2747, -28.4604)
  point P195 (33.4306, -29.2053)
  point P196 (28.9007, -24.7476)
  point P197 (29.7075, -25.8791)
  point P198 (30.7479, -27.9484)
  point P199 (31.7382, -31.0361)
  dimension "d2" = 75
  dimension "d11" = 360
  dimension "d13" = 5.904
  dimension "d15" = 11.808
  dimension "d16" = 17.712
  dimension "d17" = 23.616
  dimension "d18" = 29.52
  dimension "d19" = 85.5
  dimension "d22" = 360
  dimension "d24" = 5.904
  dimension "d25" = 11.808
  dimension "d26" = 17.712
  dimension "d27" = 23.616
  dimension "d28" = 29.52
  dimension "d32" = 360
  constraints: 420 end point, 14 point on line, 10 perpendicular, 4 coincident, 2 point on circle, 1 centre point, 1 equal length, 1 horizontal, 1 vertical, 1553 other
  measures "d2" diameter of A2
  measures "d13" distance of L40.start L40.end
  measures "d15" distance of L41.start L41.end
  measures "d16" distance of L42.start L42.end
  measures "d17" distance of L43.start L43.end
  measures "d18" distance of L44.start L44.end
  measures "d19" angle of L46 L45
  measures "d24" distance of L86.start L86.end
  measures "d25" distance of L87.start L87.end
  measures "d26" distance of L88.start L88.end
  measures "d27" distance of L89.start L89.end
  measures "d28" distance of L90.start L90.end
extrude "Extrusion1" add sketch "Sketch1" along normal blind 15 contours A2
extrude "Extrusion2" add sketch "Sketch1" along normal blind 15 contours S8 L103 A2 L104 S9 A0 | A0 S9 A1 S8
pattern_circular "Circular Pattern1" count 40 over 360 about axis through (0, 0, -10) along (0, 0, 1) of "Extrusion2"
sketch "Sketch2" plane through (0, 0, 15) normal (0, 0, 1) x (1, 0, 0)
  circle A0 centre (0, 0) radius 5
  dimension "d41" = 10
  constraints: 1 centre point, 1 coincident
  measures "d41" diameter of A0
extrude "Extrusion3" cut sketch "Sketch2" against normal blind 15
equation "\"d15\" = 2 * d13"
equation "\"d16\" = 3 * d13"
equation "\"d17\" = 4 * d13"
equation "\"d18\" = 5 * d13"
equation "\"d24\" = d13"
equation "\"d25\" = d15"
equation "\"d26\" = d16"
equation "\"d27\" = d17"
equation "\"d28\" = d18"
equation "\"d3\" = 0.939693 * d0"
equation "\"d0\" = 80"
body "Solid1"
